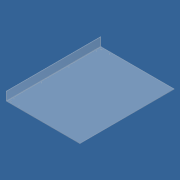
# Autodesk Inventor part: GE-12062
Saved by Autodesk Inventor 2012 (Build 160160000, 160)
## iProperties
Created: 2011-11-14
Part Number: GE-12062
Document SubType Name: Modeling
Designer: mcyr
Density: 1 g/cm^3
Description: Ball Ramp
Material: Default
Title: Ball Ramp
Author: mcyr
Autodesk Inventor part; units mm, degrees
ref_plane "YZ Plane" through (0, 0, 0) normal (1, 0, 0) x (0, 1, 0)
ref_plane "XZ Plane" through (0, 0, 0) normal (0, 1, 0) x (-1, 0, 0)
ref_plane "XY Plane" through (0, 0, 0) normal (0, 0, 1) x (1, 0, 0)
sketch "Sketch1" plane through (0, 0, 0) normal (0, 0, 1) x (1, 0, 0)
  line L0 (0, 114.3) -> (0, 4.7625)
  line L1 (4.7625, 0) -> (952.5, 0)
  line L2 (952.5, 0) -> (952.5, 6.35)
  line L3 (952.5, 6.35) -> (9.525, 6.35)
  line L4 (6.35, 9.525) -> (6.35, 114.3)
  line L5 (6.35, 114.3) -> (0, 114.3)
  arc A0 (6.35, 9.525) -> (9.525, 6.35) centre (9.525, 9.525) ccw
  arc A1 (0, 4.7625) -> (4.7625, 0) centre (4.7625, 4.7625) ccw
  point P0 (0, 0)
  dimension "d0" = 114.3
  dimension "d1" = 6.35
  dimension "d2" = 6.35
  dimension "d3" = 952.5
  dimension "d4" = 3.175
  dimension "d5" = 4.7625
  constraints: 12 end point, 4 parallel, 4 point on circle, 4 tangent, 2 centre point, 2 point on line, 1 perpendicular, 1 vertical
  measures "d0" distance of L0.start point (0, 0)
  measures "d1" distance of L4.end L0.start
  measures "d2" distance of L1.end L2.end
  measures "d3" distance of point (0, 0) L1.end
  measures "d4" radius of A0
  measures "d5" radius of A1
extrude "Extrusion1" add sketch "Sketch1" against normal blind 1219.2
hole "Hole1" at (25.4, 6.35, -76.2) direction (0, -1, 0) diameter 6.731 end through all
pattern_linear "Rectangular Pattern1" count 4 spacing 355.6 along (0, 0, -1) of "Hole1"
hole "Hole2" at (38.1, 6.35, -25.4) direction (0, -1, 0) diameter 12.7 depth 25.4 tip angle 118
pattern_linear "Rectangular Pattern2" count 2 spacing 1168.4 along (0, 0, -1) of "Hole2"
hole "Hole3" at (139.7, 6.35, -25.4) direction (0, -1, 0) diameter 4.7625 depth 25.4 tip angle 118
pattern_linear "Rectangular Pattern3" count 2 spacing 1168.4 along (0, 0, -1) of "Hole3"
body "Solid1"
